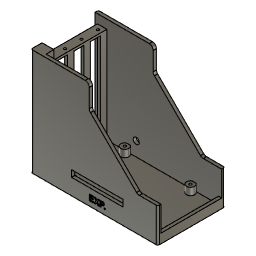
book8088_isa_exp_open_case (Autodesk Fusion 360 design; units mm, degrees)
Autodesk Fusion 360 part; units mm, degrees
sketch "스케치1" plane through (0, 0, 0) normal (0, 0, 1) x (1, 0, 0)
  line L0 (0, 75.3) -> (90.25, 75.3)
  line L1 (90.25, 75.3) -> (90.25, 0) construction
  line L2 (90.25, 0) -> (0, 0)
  line L3 (0, 0) -> (0, 75.3) construction
  line L4 (1.75, 0) -> (22.5, 0)
  line L5 (0, 1.75) -> (0, 22.5)
  line L6 (4.35, 70.95) -> (4.35, 4.35) construction
  line L7 (85.9, 70.95) -> (85.9, 4.35) construction
  line L8 (4.35, 70.95) -> (85.9, 70.95) construction
  line L9 (4.35, 4.35) -> (85.9, 4.35) construction
  circle A0 centre (4.35, 70.95) radius 1.55
  circle A1 centre (4.35, 70.95) radius 5
  circle A2 centre (85.9, 70.95) radius 1.55
  circle A3 centre (85.9, 70.95) radius 5
  circle A4 centre (85.9, 4.35) radius 1.55
  circle A5 centre (85.9, 4.35) radius 5
  circle A6 centre (4.35, 4.35) radius 1.55
  circle A7 centre (4.35, 4.35) radius 5
  line L10 (-37, 79.3) -> (120.25, 79.3)
  line L11 (120.25, 79.3) -> (120.25, -4)
  line L12 (120.25, -4) -> (-37, -4)
  line L13 (-37, -4) -> (-37, 79.3)
  line L14 (116.25, 75.3) -> (116.25, 0)
  line L15 (90.25, 75.3) -> (116.25, 75.3)
  line L16 (116.25, 0) -> (90.25, 0)
  line L17 (-34, 75.3) -> (-34, 0)
  line L18 (-34, 75.3) -> (0, 75.3)
  line L19 (-34, 0) -> (0, 0)
  line L20 (-22.25, 75.3) -> (-22.25, 0)
  line L21 (-25.75, 75.3) -> (-25.75, 0)
  line L22 (-22.25, 67.225) -> (-25.75, 67.225)
  line L23 (-25.75, 54.875) -> (-22.25, 54.875)
  line L24 (-25.75, 46.825) -> (-22.25, 46.825)
  line L25 (-25.75, 34.475) -> (-22.25, 34.475)
  line L26 (-25.75, 26.425) -> (-22.25, 26.425)
  line L27 (-22.25, 14.075) -> (-25.75, 14.075)
  line L28 (-22.25, 54.875) -> (-19.75, 54.875)
  line L29 (-19.75, 54.875) -> (-19.75, 67.225)
  line L30 (-19.75, 67.225) -> (-22.25, 67.225)
  line L31 (-22.25, 46.825) -> (-19.75, 46.825)
  line L32 (-19.75, 46.825) -> (-19.75, 34.475)
  line L33 (-19.75, 34.475) -> (-22.25, 34.475)
  line L34 (-22.25, 26.425) -> (-19.75, 26.425)
  line L35 (-19.75, 26.425) -> (-19.75, 14.075)
  line L36 (-19.75, 14.075) -> (-22.25, 14.075)
  circle A8 centre (-27.33, 69.325) radius 1.5
  line L37 (-34, 67.825) -> (-25.75, 67.825) construction
  line L38 (-25.83, 75.3) -> (-25.83, 0) construction
  line L39 (-33.7, 47.425) -> (-26.25, 47.425) construction
  circle A9 centre (-27.33, 48.925) radius 1.5
  circle A10 centre (-27.33, 28.525) radius 1.5
  line L40 (-33.7, 27.025) -> (-26.25, 27.025) construction
  line L41 (2.65, 59.35) -> (87.9, 59.35) construction
  line L42 (87.9, 59.35) -> (87.9, 50.4) construction
  line L43 (87.9, 50.4) -> (2.65, 50.4) construction
  line L44 (2.65, 50.4) -> (2.65, 59.35) construction
  line L45 (87.9, 30) -> (2.65, 30) construction
  line L46 (2.65, 38.95) -> (87.9, 38.95) construction
  line L47 (2.65, 30) -> (2.65, 38.95) construction
  line L48 (87.9, 38.95) -> (87.9, 30) construction
  line L49 (87.9, 9.6) -> (2.65, 9.6) construction
  line L50 (2.65, 18.55) -> (87.9, 18.55) construction
  line L51 (2.65, 9.6) -> (2.65, 18.55) construction
  line L52 (87.9, 18.55) -> (87.9, 9.6) construction
  line L53 (2.65, 54.875) -> (87.9, 54.875) construction
  line L54 (2.65, 34.475) -> (87.9, 34.475) construction
  line L55 (2.65, 14.075) -> (87.9, 14.075) construction
  line L56 (110.25, 59.35) -> (116.25, 59.35)
  line L57 (110.25, 50.4) -> (116.25, 50.4)
  line L58 (110.25, 59.35) -> (110.25, 56.375)
  line L59 (110.25, 56.375) -> (113.75, 56.375)
  line L60 (113.75, 56.375) -> (113.75, 53.375)
  line L61 (113.75, 53.375) -> (110.25, 53.375)
  line L62 (110.25, 53.375) -> (110.25, 50.4)
  line L63 (110.25, 38.95) -> (116.25, 38.95)
  line L64 (110.25, 38.95) -> (110.25, 35.975)
  line L65 (110.25, 35.975) -> (113.75, 35.975)
  line L66 (113.75, 35.975) -> (113.75, 32.975)
  line L67 (113.75, 32.975) -> (110.25, 32.975)
  line L68 (110.25, 32.975) -> (110.25, 30)
  line L69 (110.25, 30) -> (116.25, 30)
  line L70 (110.25, 18.55) -> (116.25, 18.55)
  line L71 (110.25, 18.55) -> (110.25, 15.575)
  line L72 (110.25, 15.575) -> (113.75, 15.575)
  line L73 (113.75, 15.575) -> (113.75, 12.575)
  line L74 (113.75, 12.575) -> (110.25, 12.575)
  line L75 (110.25, 12.575) -> (110.25, 9.6)
  line L76 (110.25, 9.6) -> (116.25, 9.6)
  line L77 (11.625, 0) -> (11.625, -4) construction
  line L78 (78.625, 0) -> (78.625, -4) construction
  line L79 (45.125, 0) -> (45.125, -4) construction
  line L80 (10.25, 79.3) -> (10.25, 75.3) construction
  line L81 (17.95, 79.3) -> (17.95, 75.3) construction
  line L82 (-37, 75.3) -> (-34, 75.3)
  line L83 (-37, 0) -> (-34, 0)
  line L84 (-22.25, 69.225) -> (-17.75, 69.225)
  line L85 (-17.75, 69.225) -> (-17.75, 52.875)
  line L86 (-17.75, 52.875) -> (-22.25, 52.875)
  line L87 (-17.75, 61.05) -> (-19.75, 61.05) construction
  line L88 (-22.25, 48.825) -> (-17.75, 48.825)
  line L89 (-17.75, 48.825) -> (-17.75, 32.475)
  line L90 (-17.75, 40.65) -> (-19.75, 40.65) construction
  line L91 (-17.75, 32.475) -> (-22.25, 32.475)
  line L92 (-22.25, 28.425) -> (-17.75, 28.425)
  line L93 (-17.75, 28.425) -> (-17.75, 12.075)
  line L94 (-17.75, 20.25) -> (-19.75, 20.25) construction
  line L95 (-17.75, 12.075) -> (-22.25, 12.075)
  line L96 (-37, 9.6) -> (-22.25, 9.6)
  line L97 (105.25, 0) -> (105.25, 7)
  line L98 (105.25, 7) -> (112.25, 7)
  line L99 (112.25, 7) -> (112.25, 0)
  circle A11 centre (108.75, 3.5) radius 3.5 construction
  circle A12 centre (108.75, 3.5) radius 1.5
  line L100 (105.25, 75.3) -> (105.25, 68.3)
  line L101 (105.25, 68.3) -> (112.25, 68.3)
  line L102 (112.25, 68.3) -> (112.25, 75.3)
  circle A13 centre (108.75, 71.8) radius 3.5 construction
  circle A14 centre (108.75, 71.8) radius 1.5
  line L103 (-12.25, 7) -> (-12.25, 0)
  line L104 (-12.25, 7) -> (-5.25, 7)
  line L105 (-5.25, 7) -> (-5.25, 0)
  line L106 (-12.25, 75.3) -> (-12.25, 68.3)
  line L107 (-12.25, 68.3) -> (-5.25, 68.3)
  line L108 (-5.25, 68.3) -> (-5.25, 75.3)
  circle A15 centre (-8.75, 71.8) radius 3.5 construction
  circle A16 centre (-8.75, 3.5) radius 3.5 construction
  circle A17 centre (-8.75, 3.5) radius 1.5
  circle A18 centre (-8.75, 71.8) radius 1.5
  dimension "d1" = 90.25
  dimension "d2" = 75.3
  dimension "d3" = 4.35
  dimension "d4" = 4.35
  dimension "d5" = 4.35
  dimension "d6" = 4.35
  dimension "d8" = 81.55
  dimension "d9" = 3.1
  dimension "d10" = 10
  dimension "d11" = 4
  dimension "d12" = 4
  dimension "d13" = 37
  dimension "d14" = 30
  dimension "d15" = 4
  dimension "d17" = 22.25
  dimension "d18" = 3.5
  dimension "d21" = 12.35
  dimension "d24" = 8.05
  dimension "d25" = 8.05
  dimension "d26" = 2.5
  dimension "d27" = 3
  dimension "d28" = 0.6
  dimension "d33" = 0.6
  dimension "d34" = 0.6
  dimension "d36" = 8.95
  dimension "d38" = 85.25
  dimension "d43" = 1.7
  dimension "d44" = 9.6
  dimension "d46" = 3
  dimension "d47" = 6
  dimension "d48" = 3.5
  dimension "d55" = 67
  dimension "d56" = 7.7
  dimension "d57" = 5.9
  dimension "d94" = 2
  dimension "d95" = 2
  dimension "d104" = 3.58
  dimension "d146" = 7
  dimension "d147" = 7
  dimension "d149" = 3
  dimension "d150" = 4
  dimension "d151" = 10
  dimension "d328" = 8.25
  constraint horizontal L0
  constraint vertical L1
  constraint horizontal L2
  constraint vertical L3
  constraint collinear L2 L4
  constraint collinear L3 L5
  constraint perpendicular L2 L6
  constraint horizontal L8
  constraint horizontal L9
  constraint equal L8 L9
  constraint equal L6 L7
  constraint perpendicular L7 L8
  constraint coincident L6 L8.start
  constraint coincident L8 L6.start
  constraint concentric A0 A1
  constraint equal A0 A2
  constraint equal A0 A6
  constraint equal A0 A4
  constraint equal A1 A3
  constraint equal A1 A7
  constraint equal A1 A5
  constraint coincident L7 L8.end
  constraint coincident L8 L7.start
  constraint coincident L7 L9.end
  constraint coincident L9 L7.end
  constraint coincident L9 L6.end
  constraint coincident L6 L9.start
  constraint concentric A2 A3
  constraint concentric A4 A5
  constraint concentric A6 A7
  constraint coincident L7.end L9.end
  constraint coincident L7.start L8.end
  constraint coincident L6.start L8.start
  constraint coincident L6.end L9.start
  constraint horizontal L10
  constraint perpendicular L10 L11
  constraint perpendicular L11 L12
  constraint perpendicular L10 L13
  constraint coincident L10.start L13.end
  constraint parallel L1 L14
  constraint perpendicular L1 L15
  constraint collinear L0 L15
  constraint coincident L0.end L1.start
  constraint coincident L14.start L15.end
  constraint horizontal L16
  constraint collinear L2 L16
  constraint coincident L1.end L2.start
  constraint coincident L14.end L16.start
  constraint perpendicular L12 L17
  constraint coincident L2.end L3.start
  constraint collinear L0 L18
  constraint collinear L2 L19
  constraint parallel L17 L20
  constraint coincident L18 L20.start
  constraint coincident L19 L20.end
  constraint parallel L20 L21
  constraint coincident L18 L21.start
  constraint coincident L19 L21.end
  constraint coincident L20 L22.start
  constraint coincident L21 L22.end
  constraint perpendicular L21 L22
  constraint coincident L21 L23.start
  constraint coincident L20 L23.end
  constraint perpendicular L20 L23
  constraint coincident L21 L24.start
  constraint coincident L20 L24.end
  constraint perpendicular L20 L24
  constraint coincident L21 L25.start
  constraint coincident L20 L25.end
  constraint perpendicular L20 L25
  constraint coincident L21 L26.start
  constraint coincident L20 L26.end
  constraint perpendicular L20 L26
  constraint coincident L20 L27.start
  constraint coincident L21 L27.end
  constraint perpendicular L21 L27
  constraint perpendicular L20 L28
  constraint perpendicular L23 L29
  constraint perpendicular L24 L32
  constraint perpendicular L26 L35
  constraint collinear L26 L34
  constraint collinear L27 L36
  constraint collinear L25 L33
  constraint collinear L24 L31
  constraint collinear L22 L30
  constraint equal L30 L31
  constraint equal L30 L34
  constraint horizontal L37
  constraint tangent A8 L37
  constraint coincident L21 L37.end
  constraint coincident L17 L37.start
  constraint vertical L38
  constraint tangent A8 L38
  constraint coincident L18 L38.start
  constraint coincident L19 L38.end
  constraint horizontal L39
  constraint tangent L39 A9
  constraint horizontal L40
  constraint tangent A10 L40
  constraint equal A8 A9
  constraint equal A8 A10
  constraint horizontal L41
  constraint vertical L42
  constraint horizontal L43
  constraint vertical L44
  constraint equal L29 L32
  constraint equal L29 L35
  constraint horizontal L46
  constraint vertical L48
  constraint horizontal L45
  constraint vertical L47
  constraint horizontal L50
  constraint vertical L52
  constraint horizontal L49
  constraint vertical L51
  constraint equal L41 L45
  constraint equal L41 L50
  constraint equal L42 L48
  constraint equal L42 L52
  constraint collinear L42 L48
  constraint collinear L42 L52
  constraint parallel L0 L53
  constraint symmetric L41 L43 L53
  constraint coincident L44 L53.start
  constraint coincident L42 L53.end
  constraint symmetric L45 L46 L54
  constraint symmetric L49 L50 L55
  constraint coincident L47 L54.start
  constraint coincident L48 L54.end
  constraint coincident L52 L55.end
  constraint coincident L51 L55.start
  constraint collinear L36 L55
  constraint collinear L33 L54
  constraint collinear L28 L53
  constraint perpendicular L1 L56
  constraint perpendicular L1 L57
  constraint equal L56 L57
  constraint collinear L41 L56
  constraint collinear L43 L57
  constraint coincident L14 L56.end
  constraint coincident L14 L57.end
  constraint perpendicular L56 L58
  constraint perpendicular L1 L59
  constraint perpendicular L59 L60
  constraint perpendicular L1 L61
  constraint perpendicular L57 L62
  constraint symmetric L53 L59 L61
  constraint equal L63 L69
  constraint perpendicular L63 L64
  constraint perpendicular L65 L66
  constraint perpendicular L68 L69
  constraint equal L70 L76
  constraint perpendicular L70 L71
  constraint perpendicular L72 L73
  constraint perpendicular L75 L76
  constraint coincident L14 L63.end
  constraint coincident L14 L69.end
  constraint coincident L14 L70.end
  constraint coincident L14 L76.end
  constraint collinear L46 L63
  constraint collinear L45 L69
  constraint collinear L50 L70
  constraint collinear L49 L76
  constraint symmetric L55 L72 L74
  constraint symmetric L54 L65 L67
  constraint perpendicular L66 L67
  constraint perpendicular L73 L74
  constraint equal L56 L63
  constraint equal L59 L65
  constraint equal L60 L66
  constraint equal L56 L70
  constraint equal L59 L72
  constraint equal L60 L73
  constraint coincident L2 L77.start
  constraint coincident L12 L77.end
  constraint perpendicular L12 L77
  constraint coincident L2 L78.start
  constraint coincident L12 L78.end
  constraint perpendicular L12 L78
  constraint coincident L2 L79.start
  constraint coincident L12 L79.end
  constraint perpendicular L12 L79
  constraint symmetric L77 L78 L79
  constraint symmetric L6 L7 L79
  constraint coincident L10 L80.start
  constraint coincident L0 L80.end
  constraint perpendicular L0 L80
  constraint coincident L10 L81.start
  constraint coincident L0 L81.end
  constraint perpendicular L0 L81
  constraint perpendicular L13 L82
  constraint collinear L18 L82
  constraint coincident L17.start L18.start
  constraint coincident L13 L82.start
  constraint horizontal L83
  constraint collinear L19 L83
  constraint coincident L17.end L19.start
  constraint coincident L13 L83.start
  constraint tangent L38 A9
  constraint tangent L38 A10
  constraint coincident L20 L84.start
  constraint perpendicular L20 L84
  constraint perpendicular L10 L85
  constraint coincident L20 L86.end
  constraint perpendicular L20 L86
  constraint coincident L85 L87.start
  constraint coincident L29 L87.end
  constraint perpendicular L29 L87
  constraint symmetric L28 L30 L87
  constraint symmetric L84 L86 L87
  constraint coincident L90.start L89
  constraint symmetric L88 L90 L91
  constraint coincident L94.start L93
  constraint symmetric L92 L94 L95
  constraint coincident L20 L88.start
  constraint coincident L32 L90.end
  constraint coincident L20 L91.end
  constraint coincident L20 L92.start
  constraint coincident L35 L94.end
  constraint coincident L20 L95.end
  constraint symmetric L34 L36 L94
  constraint symmetric L31 L33 L90
  constraint perpendicular L93 L95
  constraint perpendicular L92 L93
  constraint perpendicular L89 L91
  constraint perpendicular L88 L89
  constraint equal L87 L90
  constraint equal L87 L94
  constraint equal L85 L89
  constraint equal L85 L93
  constraint perpendicular L17 L96
  constraint collinear L49 L96
  constraint coincident L20 L96.end
  constraint coincident L13 L96.start
  constraint perpendicular L9 L97
  constraint perpendicular L97 L98
  constraint perpendicular L98 L99
  constraint coincident L2 L99.end
  constraint coincident L2 L97.start
  constraint tangent L98 A11
  constraint tangent L99 A11
  constraint tangent L97 A11
  constraint concentric A11 A12
  constraint perpendicular L8 L100
  constraint perpendicular L100 L101
  constraint perpendicular L8 L102
  constraint coincident L0 L100.start
  constraint coincident L0 L102.end
  constraint equal L98 L101
  constraint equal L99 L102
  constraint tangent L102 A13
  constraint tangent L101 A13
  constraint tangent L100 A13
  constraint concentric A13 A14
  constraint equal A12 A14
  constraint collinear L97 L100
  constraint coincident L19 L103.end
  constraint perpendicular L19 L103
  constraint perpendicular L20 L104
  constraint coincident L19 L105.end
  constraint perpendicular L19 L105
  constraint coincident L18 L106.start
  constraint perpendicular L18 L106
  constraint perpendicular L106 L107
  constraint coincident L18 L108.end
  constraint perpendicular L18 L108
  constraint equal L98 L104
  constraint equal L98 L107
  constraint equal L99 L105
  constraint equal L99 L108
  constraint collinear L103 L106
  constraint tangent L105 A16
  constraint tangent L104 A16
  constraint tangent L103 A16
  constraint tangent L108 A15
  constraint tangent L107 A15
  constraint tangent L106 A15
  constraint equal A12 A18
  constraint equal A12 A17
  constraint concentric A16 A17
  constraint concentric A15 A18
  measures "d1" distance of L1.end L2.end
  measures "d2" distance of L0.end L1.end
  measures "d3" distance of L2 L9
  measures "d4" distance of L1 L7
  measures "d5" distance of L0 L8
  measures "d6" distance of L3 L6
  measures "d8" distance of L6 L7
  measures "d9" diameter of A0
  measures "d10" diameter of A1
  measures "d11" distance of L0 L10
  measures "d12" distance of L2 L12
  measures "d13" distance of L3 L13
  measures "d14" distance of L1 L11
  measures "d15" distance of L11 L14
  measures "d17" distance of L3 L20
  measures "d18" distance of L20 L21
  measures "d21" distance of L22 L23
  measures "d24" distance of L23 L24
  measures "d25" distance of L25 L26
  measures "d26" distance of L22.start L29.end
  measures "d27" diameter of A8
  measures "d28" distance of L22 L37
  measures "d33" distance of L24 L39
  measures "d34" distance of L26 L40
  measures "d36" distance of L41.end L42.end
  measures "d38" distance of L41.start L41.end
  measures "d43" distance of L6 L44
  measures "d44" distance of L2 L49
  measures "d46" distance of L59.end L60.end
  measures "d47" distance of L56.start L56.end
  measures "d48" distance of L58.end L59.end
  measures "d55" distance of L77 L78
  measures "d56" distance of L80 L81
  measures "d57" distance of L6 L80
  measures "d94" distance of L87.start L87.end
  measures "d95" distance of L30 L84
  measures "d104" distance of L20 L38
  measures "d146" distance of L98.end L99.end
  measures "d147" distance of L97.end L98.end
  measures "d149" diameter of A12
  measures "d150" distance of L14 L102
  measures "d151" distance of L20 L103
  measures "d328" distance of L17 L21
extrude "돌출1" add sketch "스케치1" along normal blind 2.5 contours L0 L2 L4 A1 A3 A5 A7 L10 L11 L12 L13 L14 L15 L16 L18 L19 L82 L83 | L0 L2 L4 A1 A3 A5 A7 L14 L15 L16 L18 L19 L20 L56 L57 L58 L59 L60 L61 L62 L63 L64 L65 L66 L67 L68 L69 L70 L71 L72 L73 L74 L75 L76 L84 L85 L86 L88 L89 L91 L92 L93 L95 L97 L98 L99 L100 L101 L102 L103 L104 L105 L106 L107 L108 | L0 A1 | L0 A1 | L18 L106 L107 L108 | L0 A3 | L0 A3 | L18 L20 L21 L22 | L17 L18 L21 L96 | L20 L28 L29 L30 L84 L85 L86 | L13 L17 L82 L96 | L20 L21 L22 L23 | L20 L28 L29 L30 | L15 L100 L101 L102 | L17 L19 L21 L96 | L13 L17 L83 L96 | L20 L21 L23 L24 | L19 L20 L21 L96 | L20 L21 L27 L96 | L20 L21 L24 L25 | L20 L21 L26 L27 | L20 L21 L25 L26 | L20 L31 L32 L33 | L20 L31 L32 L33 L88 L89 L91 | L14 L56 L57 L58 L59 L60 L61 L62 | L20 L34 L35 L36 L92 L93 L95 | L20 L34 L35 L36 | L19 L103 L104 L105 | L14 L63 L64 L65 L66 L67 L68 L69 | L14 L70 L71 L72 L73 L74 L75 L76 | L2 L4 L5 A7 | L2 L4 A7 | L5 A7 | L16 L97 L98 L99 | L2 A5 | L2 A5 | A0 | A2 | A4 | A6 | A8 | A9 | A10 | A12 | A14 | A17 | A18
extrude "돌출2" cut sketch "스케치1" along normal through all and the other way blind 1.5 from surface at 2.5 contours L20 L28 L29 L30 | L20 L31 L32 L33 | L20 L34 L35 L36
extrude "돌출13" add sketch "스케치1" along normal blind 6.5 contours L20 L28 L29 L30 L84 L85 L86 | L20 L31 L32 L33 L88 L89 L91 | L20 L34 L35 L36 L92 L93 L95
extrude "돌출3" add sketch "스케치1" along normal blind 11.5 contours L0 A1 | L0 A1 | L0 A3 | L0 A3 | L2 L4 L5 A7 | L2 L4 A7 | L5 A7 | L2 A5 | L2 A5
extrude "돌출4" add sketch "스케치1" along normal blind 132.5 contours L0 L2 L4 A1 A3 A5 A7 L10 L11 L12 L13 L14 L15 L16 L18 L19 L82 L83 | L0 A1 | L0 A3 | L2 L4 A7 | L2 A5 picked at (4.2274, 75.722) picked at (86.0226, 75.5121) picked at (86.5, -0.1049)
extrude "돌출5" add sketch "스케치1" along normal blind 118.5 contours L18 L20 L21 L22 | L20 L21 L23 L24 | L19 L20 L21 L96 | L20 L21 L27 L96 | L20 L21 L25 L26
extrude "돌출12" add sketch "스케치1" along normal blind 21.5 contours L20 L21 L22 L23 | L20 L21 L24 L25 | L20 L21 L26 L27
extrude "돌출6" add sketch "스케치1" along normal blind 3 from surface at 118.5 contours L18 L20 L21 L22 | L17 L18 L21 L96 | L20 L21 L22 L23 | L17 L19 L21 L96 | L20 L21 L23 L24 | L19 L20 L21 L96 | L20 L21 L27 L96 | L20 L21 L24 L25 | L20 L21 L26 L27 | L20 L21 L25 L26
extrude "돌출17" add sketch "스케치1" along normal blind 132.5 contours L17 L19 L21 L96 | L13 L17 L83 L96 | L19 L20 L21 L96
extrude "돌출7" add sketch "스케치1" along normal blind 50 from surface at 31.5 contours L14 L56 L57 L58 L59 L60 L61 L62 | L14 L63 L64 L65 L66 L67 L68 L69 | L14 L70 L71 L72 L73 L74 L75 L76
chamfer "모따기9" distance 6 angle 45 3 edges at (116.25, 14.075, 81.5) (116.25, 34.475, 81.5) (116.25, 54.875, 81.5)
chamfer "모따기10" distance 6 angle 45 3 edges at (116.25, 54.875, 31.5) (116.25, 34.475, 31.5) (116.25, 14.075, 31.5)
extrude "돌출26" add sketch "스케치1" against normal blind 10 from surface at 132.5 contours L18 L106 L107 L108 | L15 L100 L101 L102 | L19 L103 L104 L105 | L16 L97 L98 L99 | A12 | A14 | A17 | A18
chamfer "모따기5" distance 7 angle 45 2 edges at (108.75, 75.3, 122.5) (-8.75, 75.3, 122.5)
chamfer "모따기6" distance 7 angle 45 2 edges at (108.75, 0, 122.5) (-8.75, 0, 122.5)
extrude "돌출27" cut sketch "스케치1" against normal blind 9 from surface at 132.5 contours A12 | A14 | A17 | A18
sketch "스케치8" plane through (0, 0, 0) normal (0, 0, -1) x (1, 0, 0)
  line L0 (-37, 4) -> (-37, -79.3)
  line L1 (-37, -79.3) -> (120.25, -79.3)
  line L2 (120.25, -79.3) -> (120.25, 4)
  line L3 (120.25, 4) -> (-37, 4)
  circle A0 centre (-22, -11) radius 10
  circle A1 centre (105.25, -11) radius 10
  circle A2 centre (105.25, -64.3) radius 10
  circle A3 centre (-22, -64.3) radius 10
  line L4 (-32, 4) -> (-32, -79.3) construction
  line L5 (115.25, 4) -> (115.25, -79.3) construction
  line L6 (-37, -1) -> (120.25, -1) construction
  line L7 (-37, -74.3) -> (120.25, -74.3) construction
  line L8 (-37, 4) -> (-37, -79.3)
  line L9 (120.25, -79.3) -> (120.25, 4)
  line L10 (120.25, 4) -> (-37, 4)
  line L11 (-37, -79.3) -> (120.25, -79.3)
  line L12 (-22, -1) -> (-22, -21)
  line L13 (-32, -11) -> (-12, -11)
  line L14 (-32, -64.3) -> (-12, -64.3)
  line L15 (-22, -54.3) -> (-22, -74.3)
  line L16 (105.25, -54.3) -> (105.25, -74.3)
  line L17 (95.25, -64.3) -> (115.25, -64.3)
  line L18 (95.25, -11) -> (115.25, -11)
  line L19 (105.25, -21) -> (105.25, -1)
  circle A4 centre (-22, -64.3) radius 8
  circle A5 centre (-22, -11) radius 8
  circle A6 centre (105.25, -11) radius 8
  circle A7 centre (105.25, -64.3) radius 8
  line L20 (-32, -12) -> (-12, -12)
  line L21 (-32, -10) -> (-12, -10)
  line L22 (-23, -1) -> (-23, -21)
  line L23 (-21, -1) -> (-21, -21)
  line L24 (-32, -65.3) -> (-12, -65.3)
  line L25 (-32, -63.3) -> (-12, -63.3)
  line L26 (-23, -54.3) -> (-23, -74.3)
  line L27 (-21, -54.3) -> (-21, -74.3)
  line L28 (95.25, -65.3) -> (115.25, -65.3)
  line L29 (95.25, -63.3) -> (115.25, -63.3)
  line L30 (104.25, -54.3) -> (104.25, -74.3)
  line L31 (106.25, -54.3) -> (106.25, -74.3)
  line L32 (95.25, -12) -> (115.25, -12)
  line L33 (95.25, -10) -> (115.25, -10)
  line L34 (106.25, -21) -> (106.25, -1)
  line L35 (104.25, -21) -> (104.25, -1)
  dimension "d218" = 5
  dimension "d219" = 5
  dimension "d220" = 5
  dimension "d221" = 5
  dimension "d222" = 20
  dimension "d223" = -2
  dimension "d224" = -2
  dimension "d225" = -2
  dimension "d226" = -2
  dimension "d227" = 1
  dimension "d228" = -1
  dimension "d229" = 1
  dimension "d230" = -1
  dimension "d231" = 1
  dimension "d232" = -1
  dimension "d233" = 1
  dimension "d234" = -1
  dimension "d235" = 1
  dimension "d236" = -1
  dimension "d237" = 1
  dimension "d238" = -1
  dimension "d239" = 1
  dimension "d240" = -1
  dimension "d241" = 1
  dimension "d242" = -1
  constraint equal A0 A1
  constraint equal A0 A2
  constraint equal A0 A3
  constraint perpendicular L3 L4
  constraint perpendicular L2 L6
  constraint horizontal L7
  constraint tangent A1 L6
  constraint tangent A1 L5
  constraint tangent A2 L5
  constraint tangent A2 L7
  constraint tangent A3 L7
  constraint tangent A3 L4
  constraint tangent A0 L4
  constraint tangent A0 L6
  constraint perpendicular L5 L6
  constraint equal L4 L5
  constraint equal L6 L7
  constraint coincident L5.start L10
  constraint coincident L5.end L11
  constraint coincident L7.end L9
  constraint coincident L6.end L9
  constraint coincident L4.start L10
  constraint coincident L7.start L8
  constraint parallel L4 L12
  constraint horizontal L14
  constraint vertical L15
  constraint vertical L16
  constraint perpendicular L18 L19
  constraint perpendicular L16 L17
  constraint perpendicular L12 L13
  constraint parallel L6 L18
  constraint coincident A1.centre L18
  constraint coincident A1.centre L19
  constraint coincident A1 L19.start
  constraint coincident A1 L19.end
  constraint coincident A1 L18.end
  constraint coincident A1 L18.start
  constraint coincident A2 L16.start
  constraint coincident A2 L16.end
  constraint coincident A2.centre L16
  constraint coincident A2.centre L17
  constraint coincident A2 L17.end
  constraint coincident A2 L17.start
  constraint coincident A3.centre L15
  constraint coincident A3.centre L14
  constraint coincident A3 L14.end
  constraint coincident A3 L14.start
  constraint coincident A3 L15.start
  constraint coincident A3 L15.end
  constraint coincident A0.centre L13
  constraint coincident A0.centre L12
  constraint coincident A0 L12.end
  constraint coincident A0 L12.start
  constraint coincident A0 L13.end
  constraint coincident A0 L13.start
  measures "d218" distance of L4 L8
  measures "d219" distance of L5 L9
  measures "d220" distance of L6 L10
  measures "d221" distance of L7 L11
  measures "d222" diameter of A0
extrude "돌출41" cut sketch "스케치8" against normal blind 0.4 contours L13 A5 L20 L23 | L13 A5 L21 L23 | L12 A5 L20 L23 | L12 A5 L20 L22 | L19 A6 L32 L34 | L19 A6 L32 L35 | L18 A6 L32 L35 | L18 A6 L33 L35 | L16 A7 L29 L31 | L16 A7 L29 L30 | L17 A7 L28 L30 | L17 A7 L29 L30 | L14 A4 L24 L27 | L14 A4 L25 L27 | L15 A4 L25 L27 | L15 A4 L25 L26
sketch "스케치7" plane through (-25.75, 0, 0) normal (-1, 0, 0) x (0, -1, 0)
  line L0 (-9.6, 2.5) -> (-9.6, 118.5)
  line L1 (-9.6, 118.5) -> (-14.075, 118.5)
  line L2 (-14.075, 118.5) -> (-14.075, 21.5)
  line L3 (-14.075, 21.5) -> (-26.425, 21.5)
  line L4 (-26.425, 21.5) -> (-26.425, 118.5)
  line L5 (-26.425, 118.5) -> (-34.475, 118.5)
  line L6 (-34.475, 118.5) -> (-34.475, 21.5)
  line L7 (-34.475, 21.5) -> (-46.825, 21.5)
  line L8 (-46.825, 21.5) -> (-46.825, 118.5)
  line L9 (-46.825, 118.5) -> (-54.875, 118.5)
  line L10 (-54.875, 118.5) -> (-54.875, 21.5)
  line L11 (-54.875, 21.5) -> (-67.225, 21.5)
  line L12 (-67.225, 21.5) -> (-67.225, 118.5)
  line L13 (-67.225, 118.5) -> (-75.3, 118.5)
  line L14 (-75.3, 118.5) -> (-75.3, 2.5)
  line L15 (-75.3, 2.5) -> (-9.6, 2.5)
  line L16 (-26.425, 7.5) -> (-14.075, 7.5) construction
  line L17 (-14.075, 7.5) -> (-14.075, 17.5) construction
  line L18 (-14.075, 17.5) -> (-26.425, 17.5) construction
  line L19 (-26.425, 17.5) -> (-26.425, 7.5) construction
  line L20 (-46.825, 7.5) -> (-34.475, 7.5) construction
  line L21 (-34.475, 7.5) -> (-34.475, 17.5) construction
  line L22 (-34.475, 17.5) -> (-46.825, 17.5) construction
  line L23 (-46.825, 17.5) -> (-46.825, 7.5) construction
  line L24 (-67.225, 7.5) -> (-54.875, 7.5) construction
  line L25 (-54.875, 7.5) -> (-54.875, 17.5) construction
  line L26 (-54.875, 17.5) -> (-67.225, 17.5) construction
  line L27 (-67.225, 17.5) -> (-67.225, 7.5) construction
  dimension "d205" = 7
  dimension "d206" = 4
  dimension "d207" = 10
  dimension "d208" = 7
  dimension "d210" = 7
  dimension "d212" = 4
  dimension "d213" = 4
  text T0 "1" font "Arial" height 7 bold align centre middle in box 12.35 x 10 at (-26.425, 7.5) x (1, 0) y (0, 1) spacing 1 kerned
  text T1 "2" font "Arial" height 7 bold align centre middle in box 12.35 x 10 at (-46.825, 7.5) x (1, 0) y (0, 1) spacing 1 kerned
  text T2 "3" font "Arial" height 7 bold align centre middle in box 12.35 x 10 at (-67.225, 7.5) x (1, 0) y (0, 1) spacing 1 kerned
  constraint collinear L4 L19
  constraint collinear L2 L17
  constraint equal L18 L22
  constraint equal L18 L26
  constraint equal L19 L23
  constraint equal L19 L27
  constraint collinear L6 L21
  constraint collinear L10 L25
  measures "d206" distance of L3 L18
  measures "d212" distance of L7 L22
  measures "d213" distance of L11 L26
extrude "돌출39" cut sketch "스케치7" against normal blind 0.5 text T0 T1 T2
sketch "Exp_Cable" plane through (0, -4, 0) normal (0, -1, 0) x (1, 0, 0)
  line L0 (-37, 0) -> (120.25, 0)
  line L1 (120.25, 0) -> (120.25, 132.5)
  line L2 (120.25, 132.5) -> (-37, 132.5)
  line L3 (-37, 132.5) -> (-37, 0)
  line L4 (11.625, 132.5) -> (11.625, 0) construction
  line L5 (78.625, 132.5) -> (78.625, 0) construction
  line L6 (-37, 13.1) -> (120.25, 13.1) construction
  line L7 (120.25, 0) -> (-37, 0)
  line L8 (13.225, 28.1) -> (77.025, 28.1)
  line L9 (77.025, 28.1) -> (77.025, 19.9)
  line L10 (77.025, 19.9) -> (13.225, 19.9)
  line L11 (13.225, 19.9) -> (13.225, 28.1)
  line L12 (11.625, 4.4) -> (78.625, 4.4) construction
  line L13 (78.625, 4.4) -> (78.625, 14.4) construction
  line L14 (78.625, 14.4) -> (11.625, 14.4) construction
  line L15 (11.625, 14.4) -> (11.625, 4.4) construction
  line L16 (78.525, 18.4) -> (11.725, 18.4)
  line L17 (11.725, 18.4) -> (11.725, 29.6)
  line L18 (11.725, 29.6) -> (78.525, 29.6)
  line L19 (78.525, 29.6) -> (78.525, 18.4)
  line L20 (45.125, 28.1) -> (45.125, 19.9) construction
  line L21 (77.025, 28.1) -> (77.025, 132.5)
  line L22 (13.225, 28.1) -> (13.225, 132.5)
  line L23 (13.225, 127.5) -> (77.025, 127.5)
  line L24 (13.225, 34.1) -> (14.625, 34.1)
  line L25 (13.225, 28.1) -> (14.625, 34.1)
  line L26 (77.025, 34.1) -> (75.625, 34.1)
  line L27 (75.625, 34.1) -> (77.025, 28.1)
  line L28 (14.625, 34.1) -> (14.625, 127.5)
  line L29 (75.625, 34.1) -> (75.625, 127.5)
  line L30 (75.625, 50.6) -> (71.225, 50.6)
  line L31 (71.225, 50.6) -> (71.225, 45.6)
  line L32 (71.225, 45.6) -> (75.625, 41.2)
  line L33 (11.625, 48.1) -> (78.625, 48.1) construction
  line L34 (14.625, 50.6) -> (19.025, 50.6)
  line L35 (19.025, 50.6) -> (19.025, 45.6)
  line L36 (19.025, 45.6) -> (14.625, 41.2)
  line L37 (14.625, 113.5) -> (75.625, 113.5) construction
  line L38 (75.625, 116) -> (71.225, 116)
  line L39 (71.225, 116) -> (71.225, 111)
  line L40 (71.225, 111) -> (75.625, 106.6)
  line L41 (14.625, 116) -> (19.025, 116)
  line L42 (19.025, 116) -> (19.025, 111)
  line L43 (19.025, 111) -> (14.625, 106.6)
  line L44 (113.25, 132.5) -> (113.25, 0) construction
  line L45 (-5.375, 127.5) -> (1.625, 127.5)
  line L46 (1.625, 127.5) -> (1.625, 19.9)
  line L47 (1.625, 19.9) -> (-5.375, 19.9)
  line L48 (-5.375, 19.9) -> (-5.375, 127.5)
  line L49 (-22.375, 127.5) -> (-15.375, 127.5)
  line L50 (-15.375, 127.5) -> (-15.375, 19.9)
  line L51 (-15.375, 19.9) -> (-22.375, 19.9)
  line L52 (-22.375, 19.9) -> (-22.375, 127.5)
  point P0 (11.625, 0)
  point P1 (78.625, 0)
  dimension "d73" = 13.1
  dimension "d74" = 8.2
  dimension "d168" = 7
  dimension "d170" = 10
  dimension "d198" = -1.5
  dimension "d286" = 6.8
  dimension "d287" = 63.8
  dimension "d312" = 5
  dimension "d317" = 6
  dimension "d318" = 1.4
  dimension "d321" = 4.4
  dimension "d322" = 5
  dimension "d323" = 20
  dimension "d331" = 19
  dimension "d332" = 4.4
  dimension "d334" = 135
  dimension "d339" = 7
  dimension "d351" = 135
  dimension "d352" = 16.5
  dimension "d393" = 7
  dimension "d394" = 10
  dimension "d398" = 10
  dimension "d420" = 4
  text T0 "EXP." font "Arial" height 7 bold align centre middle in box 67 x 10 at (11.625, 4.4) x (1, 0) y (0, 1) spacing 1 kerned
  constraint perpendicular L0 L4
  constraint coincident P0 L4.end
  constraint coincident P1 L5.end
  constraint coincident L2 L5.start
  constraint coincident L2 L4.start
  constraint perpendicular L5 L6
  constraint coincident L1 L6.end
  constraint coincident L3 L6.start
  constraint horizontal L8
  constraint vertical L9
  constraint horizontal L10
  constraint vertical L11
  constraint collinear L5 L13
  constraint collinear L4 L15
  constraint coincident L8 L20.start
  constraint coincident L10 L20.end
  constraint perpendicular L8 L20
  constraint symmetric L4 L5 L20
  constraint coincident L2 L21.end
  constraint perpendicular L2 L21
  constraint coincident L2 L22.end
  constraint perpendicular L2 L22
  constraint coincident L22 L23.start
  constraint coincident L21 L23.end
  constraint perpendicular L21 L23
  constraint perpendicular L22 L24
  constraint perpendicular L21 L26
  constraint equal L24 L26
  constraint collinear L24 L26
  constraint coincident L23 L28.end
  constraint perpendicular L23 L28
  constraint coincident L23 L29.end
  constraint perpendicular L23 L29
  constraint coincident L21 L26.start
  constraint coincident L22 L24.start
  constraint parallel L29 L31
  constraint coincident L29 L30.start
  constraint coincident L29 L32.end
  constraint coincident L4 L33.start
  constraint coincident L5 L33.end
  constraint perpendicular L5 L33
  constraint perpendicular L33 L35
  constraint coincident L28 L36.end
  constraint equal L31 L35
  constraint parallel L2 L37
  constraint coincident L29 L40.end
  constraint coincident L29 L37.end
  constraint coincident L28 L37.start
  constraint perpendicular L37 L42
  constraint coincident L28 L43.end
  constraint equal L39 L42
  constraint equal L40 L43
  constraint parallel L5 L44
  constraint coincident L2 L44.start
  constraint coincident L0 L44.end
  constraint coincident L29 L38.start
  constraint coincident L28 L41.start
  constraint vertical L39
  constraint equal L31 L39
  constraint coincident L39.end L40.start
  constraint coincident L42.end L43.start
  constraint coincident L28 L34.start
  constraint perpendicular L34 L35
  constraint perpendicular L30 L31
  constraint symmetric L30.end L31.end L33
  constraint collinear L30 L34
  constraint equal L30 L34
  constraint equal L32 L36
  constraint perpendicular L38 L39
  constraint symmetric L37 L38.end L39.end
  constraint perpendicular L41 L42
  constraint equal L38 L41
  constraint collinear L38 L41
  constraint horizontal L45
  constraint vertical L46
  constraint horizontal L47
  constraint vertical L48
  constraint collinear L10 L47
  constraint collinear L23 L45
  constraint horizontal L49
  constraint vertical L50
  constraint horizontal L51
  constraint vertical L52
  constraint equal L45 L49
  constraint collinear L45 L49
  constraint collinear L47 L51
  measures "d73" distance of L6 L7
  measures "d74" distance of L8.end L9.end
  measures "d170" distance of L12 L14
  measures "d286" distance of L6 L10
  measures "d287" distance of L9 L11
  measures "d312" distance of L2 L23
  measures "d317" distance of L8 L24
  measures "d318" distance of L22 L28
  measures "d321" distance of L29 L31
  measures "d322" distance of L30.end L31.end
  measures "d323" distance of L8 L33
  measures "d331" distance of L2 L37
  measures "d332" horizontal distance of L39.end L40.end
  measures "d334" angle of L39 L40
  measures "d339" distance of L1 L44
  measures "d351" angle of L31 L32
  measures "d352" distance of L2 L38
  measures "d393" distance of L45.start L45.end
  measures "d394" distance of L4 L46
  measures "d398" distance of L48 L50
  measures "d420" distance of L14 L16
extrude "돌출8" cut sketch "Exp_Cable" against normal blind 4 contours L8 L9 L10 L11
extrude "돌출76" cut sketch "Exp_Cable" against normal blind 0.5 text T0
sketch "스케치4" plane through (0, 79.3, 0) normal (0, 1, 0) x (-1, 0, 0)
  line L0 (-120.25, 0) -> (37, 0)
  line L1 (37, 0) -> (37, 132.5)
  line L2 (37, 132.5) -> (-120.25, 132.5)
  line L3 (-120.25, 132.5) -> (-120.25, 0)
  line L4 (-17.95, 132.5) -> (-17.95, 0) construction
  line L5 (-10.25, 132.5) -> (-10.25, 0) construction
  line L6 (-120.25, 13.1) -> (37, 13.1) construction
  line L7 (37, 0) -> (-120.25, 0)
  circle A0 centre (-14.1, 19.95) radius 3.85
  line L8 (-17.95, 16.1) -> (-10.25, 16.1) construction
  line L9 (-106, 13.1) -> (34, 13.1)
  line L10 (34, 13.1) -> (34, 11.6)
  line L11 (34, 11.6) -> (-106, 11.6)
  line L12 (-106, 11.6) -> (-106, 13.1)
  line L13 (-9.25, 14.95) -> (4.75, 14.95) construction
  line L14 (4.75, 14.95) -> (4.75, 24.95) construction
  line L15 (4.75, 24.95) -> (-9.25, 24.95) construction
  line L16 (-9.25, 24.95) -> (-9.25, 14.95) construction
  line L17 (-17.95, 19.95) -> (-10.25, 19.95) construction
  line L18 (-70, 43.1) -> (30, 43.1) construction
  line L19 (30, 43.1) -> (30, 70.1) construction
  line L20 (30, 70.1) -> (-70, 70.1) construction
  line L21 (-70, 70.1) -> (-70, 43.1) construction
  point P0 (-10.25, 0)
  point P1 (-17.95, 0)
  dimension "d78" = 13.1
  dimension "d82" = 3
  dimension "d177" = 1.5
  dimension "d178" = 3
  dimension "d180" = 3
  dimension "d183" = 4
  dimension "d184" = 1
  dimension "d185" = 14
  dimension "d187" = 10
  dimension "d190" = 9
  dimension "d309" = 14.25
  dimension "d425" = 27
  dimension "d426" = 100
  dimension "d427" = 7
  dimension "d428" = 30
  text T0 "DC 12V" font "Arial" height 4 bold align centre middle in box 14 x 10 at (-9.25, 14.95) x (1, 0) y (0, 1) spacing 1 kerned
  text T1 "Book8088\nISA EXPANSION" font "Arial" height 9 bold align centre middle in box 100 x 27 at (-70, 43.1) x (1, 0) y (0, 1) spacing 1 kerned
  constraint vertical L4
  constraint vertical L5
  constraint coincident P0 L5.end
  constraint coincident P1 L4.end
  constraint coincident L2 L5.start
  constraint coincident L2 L4.start
  constraint horizontal L6
  constraint coincident L1 L6.end
  constraint coincident L3 L6.start
  constraint tangent L4 A0
  constraint tangent L5 A0
  constraint perpendicular L4 L8
  constraint coincident L5 L8.end
  constraint coincident L4 L8.start
  constraint tangent A0 L8
  constraint horizontal L9
  constraint vertical L10
  constraint horizontal L11
  constraint vertical L12
  constraint perpendicular L4 L17
  constraint coincident L4 L17.start
  constraint coincident L5 L17.end
  constraint coincident A0.centre L17
  constraint horizontal L18
  measures "d78" distance of L6 L7
  measures "d82" distance of L6 L8
  measures "d177" distance of L9 L11
  measures "d178" distance of L8 L9
  measures "d180" distance of L1 L10
  measures "d184" distance of L5 L16
  measures "d309" distance of L3 L12
  measures "d427" distance of L1 L19
  measures "d428" distance of L6 L18
extrude "돌출9" cut sketch "스케치4" against normal blind 4 contours A0
extrude "돌출34" cut sketch "스케치4" against normal blind 0.5 contours L9 L10 L11 L12
chamfer "모따기8" distance 0.5 angle 45 1 edges at (36, 78.8, 11.6)
extrude "돌출35" cut sketch "스케치4" against normal blind 0.5 text T0
sketch "스케치13" plane through (120.25, 0, 0) normal (1, 0, 0) x (0, 1, 0)
  line L0 (-4, 0) -> (79.3, 0)
  line L1 (79.3, 0) -> (79.3, 132.5)
  line L2 (79.3, 132.5) -> (-4, 132.5)
  line L3 (-4, 132.5) -> (-4, 0)
  line L4 (0, 132.5) -> (75.3, 132.5)
  line L5 (75.3, 132.5) -> (75.3, 16.5)
  line L6 (75.3, 16.5) -> (0, 16.5)
  line L7 (0, 16.5) -> (0, 132.5)
  dimension "d402" = 16.5
  dimension "d403" = 4
  dimension "d404" = 4
  constraint horizontal L4
  constraint vertical L5
  constraint horizontal L6
  constraint vertical L7
  constraint coincident L2 L4.start
  measures "d402" distance of L0 L6
  measures "d403" distance of L1 L5
  measures "d404" distance of L3 L7
extrude "돌출73" cut sketch "스케치13" against normal blind 60 contours L2 L4 L5 L6 L7
sketch "스케치12" plane through (0, 0, 132.5) normal (0, 0, 1) x (-1, 0, 0)
  circle A0 centre (8.75, -3.5) radius 1.5
  line L0 (-120.25, 0) -> (5.25, 0)
  line L1 (5.25, 0) -> (5.25, -7)
  line L2 (5.25, -7) -> (12.25, -7)
  line L3 (12.25, -7) -> (12.25, 0)
  line L4 (12.25, 0) -> (22.25, 0)
  line L5 (22.25, 0) -> (22.25, -9.6)
  line L6 (22.25, -9.6) -> (37, -9.6)
  line L7 (37, -9.6) -> (37, 4)
  line L8 (37, 4) -> (-120.25, 4)
  line L9 (-120.25, 4) -> (-120.25, 0)
  line L10 (-35.25, -79.3) -> (-120.25, -79.3)
  line L11 (-120.25, -79.3) -> (-120.25, 4)
  line L12 (-120.25, 4) -> (-35.25, 4)
  line L13 (-35.25, 4) -> (-35.25, -79.3)
  line L14 (-120.25, -79.3) -> (37, -79.3)
  line L15 (-120.25, -75.3) -> (-120.25, 0)
  line L16 (14.75, -75.3) -> (-35.25, -75.3)
  line L17 (-35.25, -75.3) -> (-35.25, 0)
  line L18 (-35.25, 0) -> (14.75, 0)
  line L19 (14.75, 0) -> (14.75, -75.3)
  dimension "d407" = 85
  dimension "d408" = 50
  dimension "d409" = 4
  dimension "d410" = 4
  constraint horizontal L10
  constraint vertical L11
  constraint horizontal L12
  constraint vertical L13
  constraint collinear L10 L14
  constraint collinear L8 L12
  constraint collinear L11 L15
  constraint horizontal L16
  constraint vertical L17
  constraint horizontal L18
  constraint vertical L19
  constraint collinear L13 L17
  measures "d407" distance of L11 L13
  measures "d408" distance of L13 L19
  measures "d409" distance of L14 L16
  measures "d410" distance of L8 L18
extrude "돌출74" cut sketch "스케치12" against normal blind 30 contours L0 L1 L2 L3 L4 L13 L16 L17 L18 L19
extrude "돌출75" cut sketch "스케치12" against normal blind 90 contours L0 L8 L9 L11 L12 L13 | L0 L10 L11 L13 L14 L15 L17
chamfer "모따기27" distance 60 angle 45 2 edges at (35.25, -2, 42.5) (35.25, 77.3, 42.5)
fillet "모깎기6" radius 2 4 edges at (120.25, 79.3, 21.25) (120.25, -4, 21.25) (-37, 79.3, 66.25) (-37, -4, 66.25)
fillet "모깎기7" radius 5 6 edges at (35.25, -2, 132.5) (35.25, -2, 102.5) (35.25, 77.3, 102.5) (35.25, 77.3, 132.5) (95.25, -2, 42.5) (95.25, 77.3, 42.5)
extrude "돌출77" cut sketch "스케치4" against normal blind 0.5 text T1
extrude "돌출78" cut sketch "스케치12" against normal blind 30 contours A0 | L0 L1 L2 L3 L4 L13 L16 L17 L18 L19 | L1 L2 L3 L18
extrude "돌출79" cut 1 faces at (118.9167, 50.2, 16.5) along direction (0, 0, -1) blind 5
equation "d3 = CARD_HOLES"
equation "d4 = CARD_HOLES"
equation "d5 = CARD_HOLES"
equation "d6 = CARD_HOLES"
equation "CARD_HOLES = 4.35 mm"
equation "d11 = CASE_WALL_OUTER_SIZE"
equation "d12 = CASE_WALL_OUTER_SIZE"
equation "d14 = CASE_WIDTH_FOR_CARD"
equation "d15 = CASE_WALL_OUTER_SIZE"
equation "SLOT_WIDTH = 12.35 mm"
equation "SLOT_GAP = 8.05 mm"
equation "d21 = SLOT_WIDTH"
equation "d24 = SLOT_GAP"
equation "d25 = SLOT_GAP"
equation "d28 = HOLE_GAP"
equation "HOLE_GAP = 0.6 mm"
equation "d33 = HOLE_GAP"
equation "d34 = HOLE_GAP"
equation "CASE_WALL_OUTER_SIZE = 4 mm"
equation "d36 = CONNECTOR_WIDTH"
equation "CONNECTOR_WIDTH = 8.95 mm"
equation "d44 = CONNECTER_GAP"
equation "CONNECTER_GAP = 9.6 mm"
equation "d58 = CASE_BOTTOM_HEIGHT"
equation "d60 = CASE_BOTTOM_HEIGHT"
equation "d62 = MOUNTING_HOLE_HEIGHT"
equation "d64 = CASE_BOTTOM_WALL_HEIGHT"
equation "d66 = SLOT_HEIGHT"
equation "d68 = SLOT_HEIGHT"
equation "d73 = MOUNTING_HOLE_GAP"
equation "d75 = -( CASE_WALL_OUTER_SIZE )"
equation "MOUNTING_HOLE_GAP = MOUNTING_HOLE_HEIGHT + 1.6 mm"
equation "d78 = MOUNTING_HOLE_GAP"
equation "d79 = -( CASE_WALL_OUTER_SIZE )"
equation "SLOT_HEIGHT = CASE_BOTTOM_HEIGHT + 116 mm"
equation "MOUNTING_HOLE_HEIGHT = CASE_BOTTOM_HEIGHT + 9 mm"
equation "SLOT_BOTTOM_HEIGHT = CASE_BOTTOM_HEIGHT + 19 mm"
equation "d90 = SLOT_BOTTOM_HEIGHT"
equation "CASE_BOTTOM_HEIGHT = 2.5 mm"
equation "CASE_BOTTOM_WALL_HEIGHT = CASE_BOTTOM_HEIGHT + 130 mm"
equation "d98 = CASE_BOTTOM_HEIGHT + 4 mm"
equation "d114 = CASE_BOTTOM_WALL_HEIGHT"
equation "d152 = CASE_BOTTOM_WALL_HEIGHT"
equation "d157 = CASE_BOTTOM_WALL_HEIGHT"
equation "d190 = CASE_CHAR_SIZE_FOR_CARD"
equation "Tolerance = 0.1 mm"
equation "d282 = MOUNTING_HOLE_HEIGHT + 20 mm"
equation "CASE_WIDTH_FOR_CARD = 30 mm"
equation "CASE_CHAR_SIZE_FOR_CARD = 9 mm"
equation "d402 = MOUNTING_HOLE_HEIGHT + 5 mm"
equation "d403 = CASE_WALL_OUTER_SIZE"
equation "d404 = CASE_WALL_OUTER_SIZE"
equation "d409 = CASE_WALL_OUTER_SIZE"
equation "d410 = CASE_WALL_OUTER_SIZE"
named bodies: "Base"
